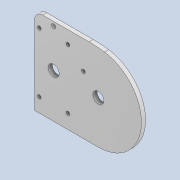
# Autodesk Inventor part: 外側フレーム
Saved by Autodesk Inventor 2020.4 (Build 244396000, 396)
## iProperties
Created: 2021-04-23
Part Number: 外側フレーム
Material: アルミニウム 2014-T4
Document SubType Name: Modeling
Designer: happy
Density: 2.8 g/cm^3
Appearance: サテン
Author: happy
Autodesk Inventor part; units mm, degrees
ref_plane "YZ Plane" through (0, 0, 0) normal (1, 0, 0) x (0, 1, 0)
ref_plane "XZ Plane" through (0, 0, 0) normal (0, 1, 0) x (-1, 0, 0)
ref_plane "XY Plane" through (0, 0, 0) normal (0, 0, 1) x (1, 0, 0)
sketch "スケッチ1" plane through (0, 0, 0) normal (0, 0, 1) x (1, 0, 0)
  circle A0 centre (96.1098, 17.5902) radius 9.025 construction
  circle A1 centre (128.7687, 16.8502) radius 6.025 construction
  line L0 (78.0196, 48.6804) -> (110.2, 48.6804) construction
  line L1 (127.2, -14.5) -> (65.0196, -14.5)
  circle A2 centre (80.0196, 33.6804) radius 15 construction
  line L2 (65.0196, -14.5) -> (65.0196, 33.6804) construction
  circle A3 centre (96.1098, 17.5902) radius 5.0587 construction
  circle A4 centre (128.7687, 16.8502) radius 29.3819 construction
  circle A5 centre (128.7687, 16.8502) radius 31.3502
  arc A6 (102.5247, 30.0621) -> (101.9533, 4.8405) centre (96.1098, 17.5902) ccw
  line L3 (88.0848, 48.6804) -> (121.9521, 48.6804)
  arc A7 (133.1613, 47.8912) -> (121.9521, 48.6804) centre (121.9521, -31.3196) ccw
  arc A8 (88.0848, 48.6804) -> (82.0848, 42.6804) centre (88.0848, 42.6804) ccw
  line L4 (82.0848, 42.6804) -> (82.0848, -14.5)
  circle A9 centre (96.1098, 17.5902) radius 4.025
  circle A10 centre (128.7687, 16.8502) radius 4.025
  line L5 (127.2, -14.5) -> (128.7687, -14.5)
  circle A11 centre (68.0196, 17.5902) radius 1.5
  circle A12 centre (96.1098, 45.6804) radius 1.5
  circle A13 centre (74.3628, 28.0235) radius 1.3
  circle A14 centre (85.6765, 39.3372) radius 1.3
  circle A15 centre (106.5431, 39.3372) radius 1.3
  circle A16 centre (117.8569, 28.0235) radius 1.3
  circle A17 centre (117.8569, 7.1569) radius 1.3
  circle A18 centre (106.5431, -4.1569) radius 1.3
  circle A19 centre (85.6765, -4.1569) radius 1.3
  circle A20 centre (74.3628, 7.1569) radius 1.3
  point P0 (0, 0)
  point P1 (0, 0)
  dimension "d0" = 5
  dimension "d1" = 80
  dimension "d2" = 6
  dimension "d3" = 8.05
  dimension "d4" = 8.05
  dimension "d7" = 3
  dimension "d8" = 3
  dimension "d9" = 2.6
  dimension "d10" = 16
  constraints: 20 centre point, 12 end point, 10 point on circle, 7 equal radius, 6 tangent, 4 coincident, 4 horizontal, 2 point on line, 1 perpendicular, 16 other
  measures "d0" radial gap between concentric circles of A0 A6
  measures "d1" radius of A7
  measures "d2" radius of A8
  measures "d3" diameter of A9
  measures "d4" diameter of A10
  measures "d7" diameter of A11
  measures "d8" diameter of A12
  measures "d9" diameter of A13
  measures "d10" distance of A14.centre A13.centre
extrude "押し出し1" add sketch "スケッチ1" along normal blind 3 contours L1 L4 A6 A5 A18 L5 | A5 A18 A9 A15 | L4 A8 L3 A7 A5 A15 A6 | A6 A5 A9 | A17
